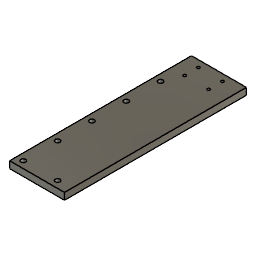
cover rolls mount left (Autodesk Fusion 360 design; units mm, degrees)
Autodesk Fusion 360 part; units mm, degrees
sketch "Szkic1" plane through (0, 0, 0) normal (0, 0, 1) x (1, 0, 0)
  circle A0 centre (-15, -15) radius 2
  circle A1 centre (-15, 5) radius 2
  circle A2 centre (20, 5) radius 2
  circle A3 centre (-15, 5) radius 2
  line L0 (-35, 0) -> (-35, 15)
  line L1 (-10, -40) -> (-35, -40)
  circle A4 centre (20, -15) radius 2
  line L2 (-35, -40) -> (35, -40)
  circle A5 centre (-15, -15) radius 2
  line L3 (-35, 15) -> (-10, 15)
  line L4 (35, -40) -> (35, 15)
  line L5 (-35, -40) -> (-35, 0)
  line L6 (-35, 15) -> (-35, -40)
  line L7 (35, 15) -> (-35, 15)
  line L8 (-10, 15) -> (-10, -40)
  line L9 (-35, -40) -> (-35, -250)
  line L10 (35, -40) -> (35, -250)
  line L11 (-35, -250) -> (35, -250)
  circle A6 centre (-25, -240) radius 1.75
  circle A7 centre (25, -240) radius 1.75
  circle A8 centre (-25, -190) radius 1.75
  circle A9 centre (-25, -140) radius 1.75
  circle A10 centre (-25, -90) radius 1.75
  circle A11 centre (-25, -40) radius 1.75
  dimension "d10" = 4
  dimension "d11" = 4
  dimension "d12" = 4
  dimension "d13" = 210
  dimension "d14" = 210
  dimension "d15" = 3.5
  dimension "d16" = 3.5
  dimension "d17" = 3.5
  dimension "d18" = 3.5
  dimension "d19" = 3.5
  dimension "d20" = 3.5
  constraint perpendicular L2 L4
  constraint parallel L2 L7
  constraint parallel L4 L6
  constraint perpendicular L2 L8
  constraint coincident L1.end L2.start
  constraint concentric A1 A3
  constraint concentric A0 A5
  constraint perpendicular L2 L9
  constraint perpendicular L2 L10
  constraint coincident L1 A11.centre
  measures "d10" diameter of A0
  measures "d11" diameter of A4
  measures "d12" diameter of A2
  measures "d13" distance of L1.end L9.end
  measures "d14" distance of L2.end L10.end
  measures "d15" diameter of A6
  measures "d16" diameter of A7
  measures "d17" diameter of A8
  measures "d18" diameter of A9
  measures "d19" diameter of A10
  measures "d20" diameter of A11
extrude "Wyciągnięcie proste1" add sketch "Szkic1" along normal blind 10 contours L0 L1 L2 L3 L5 L6 L7 L8 A11 | L1 L2 L9 L10 L11 A11 | L2 L4 L7 L8
extrude "Wyciągnięcie proste2" add 2 faces at (35, -110, 6.6667) (35, -21.6667, 3.3333) along direction (1, 0, 0) blind 10
sketch "Szkic2" plane through (0, 0, 0) normal (0, 0, -1) x (1, 0, 0)
  circle A0 centre (-25, 240) radius 1.75
  circle A1 centre (-25, 190) radius 1.75
  circle A2 centre (-25, 40) radius 1.75
  circle A3 centre (25, 240) radius 1.75
  circle A4 centre (20, -5) radius 2
  circle A5 centre (-25, 90) radius 1.75
  circle A6 centre (-15, 15) radius 2
  circle A7 centre (-25, 140) radius 1.75
  circle A8 centre (-15, -5) radius 2
  circle A9 centre (20, 15) radius 2
  line L0 (45, 250) -> (-35, 250)
  line L1 (-35, 250) -> (-35, -15)
  line L2 (-35, -15) -> (45, -15)
  line L3 (45, -15) -> (45, 250)
  circle A10 centre (-15, -5) radius 3.5
  circle A11 centre (20, -5) radius 3.5
  circle A12 centre (-15, 15) radius 3.5
  circle A13 centre (20, 15) radius 3.5
  dimension "d25" = 7
  dimension "d26" = 7
  dimension "d27" = 7
  dimension "d28" = 7
  constraint concentric A8 A10
  constraint concentric A4 A11
  constraint concentric A6 A12
  constraint concentric A9 A13
  measures "d25" diameter of A10
  measures "d26" diameter of A11
  measures "d27" diameter of A12
  measures "d28" diameter of A13
extrude "Wyciągnięcie proste3" cut sketch "Szkic2" against normal blind 5 contours A10 | A11 | A12 | A13
sketch "Szkic3" plane through (0, 0, 10) normal (0, 0, 1) x (-1, 0, 0)
  circle A0 centre (25, 240) radius 1.75
  circle A1 centre (25, 190) radius 1.75
  circle A2 centre (25, 40) radius 1.75
  circle A3 centre (-25, 240) radius 1.75
  circle A4 centre (-20, -5) radius 2
  circle A5 centre (25, 90) radius 1.75
  circle A6 centre (15, 15) radius 2
  circle A7 centre (25, 140) radius 1.75
  circle A8 centre (15, -5) radius 2
  circle A9 centre (-20, 15) radius 2
  line L0 (-45, -15) -> (35, -15)
  line L1 (35, -15) -> (35, 250)
  line L2 (35, 250) -> (-45, 250)
  line L3 (-45, 250) -> (-45, -15)
  circle A10 centre (-25, 240) radius 3.5
  circle A11 centre (25, 240) radius 3.5
  circle A12 centre (25, 190) radius 3.5
  circle A13 centre (25, 140) radius 3.5
  circle A14 centre (25, 90) radius 3.5
  circle A15 centre (25, 40) radius 3.5
  dimension "d31" = 7
  dimension "d32" = 7
  dimension "d33" = 7
  dimension "d34" = 7
  dimension "d35" = 7
  dimension "d36" = 7
  constraint concentric A3 A10
  constraint concentric A0 A11
  constraint concentric A1 A12
  constraint concentric A7 A13
  constraint concentric A5 A14
  constraint concentric A2 A15
  measures "d31" diameter of A10
  measures "d32" diameter of A11
  measures "d33" diameter of A12
  measures "d34" diameter of A13
  measures "d35" diameter of A14
  measures "d36" diameter of A15
extrude "Wyciągnięcie proste4" cut sketch "Szkic3" against normal blind 5 contours A10 | A11 | A12 | A13 | A14 | A15
